Autodesk Fusion 360 part; units mm, degrees
(part 9 of 18)
  spline S49 degree 5 poles (-11.2929, 31.6454) (-11.2932, 31.6412) (-11.294, 31.6329) (-11.2951, 31.6204) (-11.2966, 31.6038) (-11.2984, 31.5831) (-11.3001, 31.5624) (-11.3019, 31.5417) (-11.3036, 31.5211) (-11.3052, 31.5006) (-11.3069, 31.48) (-11.3085, 31.4595) (-11.31, 31.4391) (-11.3116, 31.4187) (-11.3131, 31.3983) (-11.3145, 31.378) (-11.3159, 31.3577) (-11.3173, 31.3375) (-11.3187, 31.3173) (-11.32, 31.2971) (-11.3213, 31.277) (-11.3226, 31.2569) (-11.3238, 31.2369) (-11.325, 31.2169) (-11.3262, 31.1969) (-11.3273, 31.177) (-11.3284, 31.1572) (-11.3294, 31.1374) (-11.3305, 31.1176) (-11.3315, 31.0979) (-11.3324, 31.0782) (-11.3334, 31.0585) (-11.3343, 31.0389) (-11.3351, 31.0194) (-11.336, 30.9999) (-11.3368, 30.9804) (-11.3375, 30.961) (-11.3383, 30.9416) (-11.339, 30.9223) (-11.3397, 30.903) (-11.3403, 30.8838) (-11.3409, 30.8646) (-11.3415, 30.8455) (-11.342, 30.8264) (-11.3426, 30.8073) (-11.343, 30.7884) (-11.3435, 30.7694) (-11.3439, 30.7505) (-11.3443, 30.7316) (-11.3447, 30.7128) (-11.345, 30.6941) (-11.3453, 30.6754) (-11.3456, 30.6567) (-11.3458, 30.6381) (-11.3461, 30.6195) (-11.3462, 30.601) (-11.3464, 30.5826) (-11.3465, 30.5642) (-11.3466, 30.5458) (-11.3467, 30.5275) (-11.3467, 30.5092) (-11.3467, 30.491) (-11.3467, 30.4728) (-11.3466, 30.4547) (-11.3466, 30.4367) (-11.3464, 30.4187) (-11.3463, 30.4007) (-11.3461, 30.3828) (-11.3459, 30.365) (-11.3457, 30.3472) (-11.3455, 30.3294) (-11.3452, 30.3117) (-11.3449, 30.2941) (-11.3445, 30.2765) (-11.3442, 30.259) (-11.3438, 30.2415) (-11.3434, 30.2241) (-11.3429, 30.2067) (-11.3424, 30.1894) (-11.3419, 30.1722) (-11.3414, 30.155) (-11.3409, 30.1378) (-11.3403, 30.1207) (-11.3397, 30.1037) (-11.339, 30.0867) (-11.3384, 30.0698) (-11.3377, 30.053) (-11.337, 30.0362) (-11.3363, 30.0194) (-11.3355, 30.0027) (-11.3347, 29.9861) (-11.3339, 29.9695) (-11.3331, 29.953) (-11.3322, 29.9366) (-11.3313, 29.9202) (-11.3304, 29.9038) (-11.3295, 29.8876) (-11.3285, 29.8714) (-11.3275, 29.8552) (-11.3265, 29.8391) (-11.3255, 29.8231) (-11.3244, 29.8071) (-11.3234, 29.7912) (-11.3222, 29.7754) (-11.3211, 29.7596) (-11.32, 29.7439) (-11.3188, 29.7282) (-11.3176, 29.7126) (-11.3164, 29.6971) (-11.3152, 29.6817) (-11.3139, 29.6663) (-11.3126, 29.6509) (-11.3113, 29.6357) (-11.31, 29.6205) (-11.3087, 29.6053) (-11.3073, 29.5903) (-11.3059, 29.5753) (-11.3045, 29.5603) (-11.3031, 29.5454) (-11.3016, 29.5306) (-11.3002, 29.5159) (-11.2987, 29.5013) (-11.2972, 29.4867) (-11.2957, 29.4721) (-11.2941, 29.4577) (-11.2926, 29.4433) (-11.291, 29.429) (-11.2894, 29.4147) (-11.2878, 29.4006) (-11.2861, 29.3865) (-11.2845, 29.3724) (-11.2828, 29.3585) (-11.2811, 29.3446) (-11.2794, 29.3308) (-11.2777, 29.317) (-11.276, 29.3034) (-11.2742, 29.2898) (-11.2725, 29.2763) (-11.2707, 29.2628) (-11.2689, 29.2495) (-11.2671, 29.2362) (-11.2653, 29.223) (-11.2634, 29.2098) (-11.2616, 29.1968) (-11.2597, 29.1838) (-11.2578, 29.1709) (-11.2559, 29.1581) (-11.254, 29.1453) (-11.2521, 29.1327) (-11.2502, 29.1201) (-11.2482, 29.1076) (-11.2463, 29.0952) (-11.2443, 29.0829) (-11.2423, 29.0706) (-11.2403, 29.0584) (-11.2383, 29.0464) (-11.2363, 29.0344) (-11.2343, 29.0224) (-11.2323, 29.0106) (-11.2302, 28.9989) (-11.2282, 28.9872) (-11.2261, 28.9756) (-11.2241, 28.9642) (-11.222, 28.9528) (-11.2199, 28.9415) (-11.2179, 28.9302) (-11.2158, 28.9191) (-11.2137, 28.9081) (-11.2116, 28.8971) (-11.2095, 28.8863) (-11.2074, 28.8755) (-11.2053, 28.8649) (-11.2032, 28.8543) (-11.201, 28.8438) (-11.1989, 28.8335) (-11.1968, 28.8232) (-11.1947, 28.813) (-11.1926, 28.8029) (-11.1904, 28.7929) (-11.1883, 28.783) (-11.1862, 28.7733) (-11.1841, 28.7636) (-11.1819, 28.754) (-11.1798, 28.7445) (-11.1777, 28.7351) (-11.1756, 28.7259) (-11.1735, 28.7167) (-11.1714, 28.7076) (-11.1693, 28.6987) (-11.1672, 28.6898) (-11.1651, 28.6811) (-11.163, 28.6725) (-11.1609, 28.6639) (-11.1588, 28.6555) (-11.1568, 28.6473) (-11.1547, 28.6391) (-11.1527, 28.631) (-11.1507, 28.6231) (-11.1486, 28.6153) (-11.1466, 28.6075) (-11.1446, 28.6) (-11.1427, 28.5925) (-11.1407, 28.5851) (-11.1387, 28.5779) (-11.1368, 28.5708) (-11.1349, 28.5639) (-11.133, 28.557) (-11.1311, 28.5503) (-11.1293, 28.5437) (-11.1274, 28.5373) (-11.1256, 28.531) (-11.1238, 28.5248) (-11.1221, 28.5187) (-11.1203, 28.5128) (-11.1186, 28.5071) (-11.1169, 28.5014) (-11.1153, 28.496) (-11.1136, 28.4906) (-11.112, 28.4854) (-11.1105, 28.4804) (-11.1089, 28.4755) (-11.1074, 28.4708) (-11.106, 28.4662) (-11.1046, 28.4618) (-11.1032, 28.4575) (-11.1018, 28.4534) (-11.1005, 28.4495) (-11.0993, 28.4457) (-11.0981, 28.4421) (-11.0969, 28.4387) (-11.0958, 28.4354) (-11.0948, 28.4323) (-11.0937, 28.4294) (-11.0928, 28.4267) (-11.0919, 28.4242) (-11.0911, 28.4219) (-11.0903, 28.4197) (-11.0896, 28.4178) (-11.089, 28.4161) (-11.0884, 28.4145) (-11.0879, 28.4132) (-11.0876, 28.4124) (-11.0874, 28.4118) (-11.0873, 28.4115) (-11.0872, 28.4113) knots -1 -1 -1 -1 -1 -1 -0.99583333 -0.99166667 -0.9875 -0.98333333 -0.97916667 -0.975 -0.97083333 -0.96666667 -0.9625 -0.95833333 -0.95416667 -0.95 -0.94583333 -0.94166667 -0.9375 -0.93333333 -0.92916667 -0.925 -0.92083333 -0.91666667 -0.9125 -0.90833333 -0.90416667 -0.9 -0.89583333 -0.89166667 -0.8875 -0.88333333 -0.87916667 -0.875 -0.87083333 -0.86666667 -0.8625 -0.85833333 -0.85416667 -0.85 -0.84583333 -0.84166667 -0.8375 -0.83333333 -0.82916667 -0.825 -0.82083333 -0.81666667 -0.8125 -0.80833333 -0.80416667 -0.8 -0.79583333 -0.79166667 -0.7875 -0.78333333 -0.77916667 -0.775 -0.77083333 -0.76666667 -0.7625 -0.75833333 -0.75416667 -0.75 -0.74583333 -0.74166667 -0.7375 -0.73333333 -0.72916667 -0.725 -0.72083333 -0.71666667 -0.7125 -0.70833333 -0.70416667 -0.7 -0.69583333 -0.69166667 -0.6875 -0.68333333 -0.67916667 -0.675 -0.67083333 -0.66666667 -0.6625 -0.65833333 -0.65416667 -0.65 -0.64583333 -0.64166667 -0.6375 -0.63333333 -0.62916667 -0.625 -0.62083333 -0.61666667 -0.6125 -0.60833333 -0.60416667 -0.6 -0.59583333 -0.59166667 -0.5875 -0.58333333 -0.57916667 -0.575 -0.57083333 -0.56666667 -0.5625 -0.55833333 -0.55416667 -0.55 -0.54583333 -0.54166667 -0.5375 -0.53333333 -0.52916667 -0.525 -0.52083333 -0.51666667 -0.5125 -0.50833333 -0.50416667 -0.5 -0.49583333 -0.49166667 -0.4875 -0.48333333 -0.47916667 -0.475 -0.47083333 -0.46666667 -0.4625 -0.45833333 -0.45416667 -0.45 -0.44583333 -0.44166667 -0.4375 -0.43333333 -0.42916667 -0.425 -0.42083333 -0.41666667 -0.4125 -0.40833333 -0.40416667 -0.4 -0.39583333 -0.39166667 -0.3875 -0.38333333 -0.37916667 -0.375 -0.37083333 -0.36666667 -0.3625 -0.35833333 -0.35416667 -0.35 -0.34583333 -0.34166667 -0.3375 -0.33333333 -0.32916667 -0.325 -0.32083333 -0.31666667 -0.3125 -0.30833333 -0.30416667 -0.3 -0.29583333 -0.29166667 -0.2875 -0.28333333 -0.27916667 -0.275 -0.27083333 -0.26666667 -0.2625 -0.25833333 -0.25416667 -0.25 -0.24583333 -0.24166667 -0.2375 -0.23333333 -0.22916667 -0.225 -0.22083333 -0.21666667 -0.2125 -0.20833333 -0.20416667 -0.2 -0.19583333 -0.19166667 -0.1875 -0.18333333 -0.17916667 -0.175 -0.17083333 -0.16666667 -0.1625 -0.15833333 -0.15416667 -0.15 -0.14583333 -0.14166667 -0.1375 -0.13333333 -0.12916667 -0.125 -0.12083333 -0.11666667 -0.1125 -0.10833333 -0.10416667 -0.1 -0.09583333 -0.09166667 -0.0875 -0.08333333 -0.07916667 -0.075 -0.07083333 -0.06666667 -0.0625 -0.05833333 -0.05416667 -0.05 -0.04583333 -0.04166667 -0.0375 -0.03333333 -0.02916667 -0.025 -0.02083333 -0.01666667 -0.0125 -0.00833333 -0.00416667 0 0 0 0 0 0
  line L98 (-11.0872, 28.4113) -> (-11.0867, 28.41)
  line L99 (-11.0867, 28.41) -> (-10.4972, 26.8993)
  arc A50 (-10.4972, 26.8993) -> (-12.9661, 25.8001) centre (0, 0) ccw
  line L100 (-12.9661, 25.8001) -> (-13.6943, 27.2491)
  line L101 (-13.6943, 27.2491) -> (-13.6949, 27.2503)
  spline S50 degree 5 poles (-13.6949, 27.2503) (-13.695, 27.2504) (-13.6952, 27.2507) (-13.6954, 27.2513) (-13.6959, 27.2521) (-13.6965, 27.2533) (-13.6973, 27.2548) (-13.6981, 27.2564) (-13.6991, 27.2582) (-13.7002, 27.2602) (-13.7014, 27.2624) (-13.7026, 27.2647) (-13.704, 27.2673) (-13.7055, 27.2699) (-13.7071, 27.2728) (-13.7087, 27.2758) (-13.7105, 27.2789) (-13.7124, 27.2823) (-13.7144, 27.2857) (-13.7164, 27.2893) (-13.7186, 27.293) (-13.7208, 27.2969) (-13.7231, 27.3009) (-13.7256, 27.3051) (-13.7281, 27.3094) (-13.7307, 27.3138) (-13.7334, 27.3183) (-13.7362, 27.323) (-13.7391, 27.3278) (-13.742, 27.3327) (-13.7451, 27.3377) (-13.7482, 27.3428) (-13.7514, 27.3481) (-13.7547, 27.3534) (-13.7581, 27.3589) (-13.7616, 27.3645) (-13.7652, 27.3701) (-13.7688, 27.3759) (-13.7726, 27.3818) (-13.7764, 27.3878) (-13.7803, 27.3939) (-13.7843, 27.4001) (-13.7883, 27.4063) (-13.7925, 27.4127) (-13.7967, 27.4192) (-13.801, 27.4257) (-13.8054, 27.4324) (-13.8098, 27.4391) (-13.8144, 27.446) (-13.819, 27.4529) (-13.8237, 27.4599) (-13.8285, 27.4669) (-13.8334, 27.4741) (-13.8383, 27.4813) (-13.8433, 27.4887) (-13.8484, 27.4961) (-13.8536, 27.5035) (-13.8588, 27.5111) (-13.8641, 27.5187) (-13.8695, 27.5264) (-13.875, 27.5342) (-13.8806, 27.542) (-13.8862, 27.55) (-13.8919, 27.558) (-13.8977, 27.566) (-13.9035, 27.5741) (-13.9095, 27.5823) (-13.9155, 27.5906) (-13.9215, 27.5989) (-13.9277, 27.6073) (-13.9339, 27.6158) (-13.9402, 27.6243) (-13.9466, 27.6329) (-13.953, 27.6415) (-13.9595, 27.6502) (-13.9661, 27.659) (-13.9727, 27.6678) (-13.9795, 27.6767) (-13.9863, 27.6856) (-13.9931, 27.6946) (-14.0001, 27.7037) (-14.0071, 27.7128) (-14.0142, 27.7219) (-14.0213, 27.7311) (-14.0286, 27.7404) (-14.0359, 27.7497) (-14.0432, 27.7591) (-14.0507, 27.7685) (-14.0582, 27.778) (-14.0657, 27.7875) (-14.0734, 27.7971) (-14.0811, 27.8067) (-14.0889, 27.8164) (-14.0967, 27.8261) (-14.1046, 27.8358) (-14.1126, 27.8456) (-14.1207, 27.8555) (-14.1288, 27.8654) (-14.137, 27.8753) (-14.1453, 27.8853) (-14.1536, 27.8954) (-14.162, 27.9054) (-14.1704, 27.9155) (-14.179, 27.9257) (-14.1876, 27.9359) (-14.1962, 27.9461) (-14.205, 27.9564) (-14.2137, 27.9667) (-14.2226, 27.9771) (-14.2315, 27.9875) (-14.2405, 27.9979) (-14.2496, 28.0084) (-14.2587, 28.0189) (-14.2679, 28.0294) (-14.2772, 28.04) (-14.2865, 28.0506) (-14.2959, 28.0613) (-14.3053, 28.0719) (-14.3148, 28.0827) (-14.3244, 28.0934) (-14.3341, 28.1042) (-14.3438, 28.115) (-14.3536, 28.1259) (-14.3634, 28.1368) (-14.3733, 28.1477) (-14.3833, 28.1586) (-14.3933, 28.1696) (-14.4034, 28.1806) (-14.4136, 28.1916) (-14.4238, 28.2027) (-14.4341, 28.2138) (-14.4444, 28.2249) (-14.4548, 28.2361) (-14.4653, 28.2473) (-14.4758, 28.2585) (-14.4864, 28.2697) (-14.4971, 28.281) (-14.5078, 28.2923) (-14.5186, 28.3036) (-14.5295, 28.3149) (-14.5404, 28.3263) (-14.5514, 28.3377) (-14.5624, 28.3491) (-14.5735, 28.3606) (-14.5847, 28.372) (-14.5959, 28.3835) (-14.6072, 28.395) (-14.6185, 28.4066) (-14.6299, 28.4181) (-14.6414, 28.4297) (-14.6529, 28.4413) (-14.6645, 28.4529) (-14.6761, 28.4646) (-14.6878, 28.4763) (-14.6996, 28.4879) (-14.7114, 28.4997) (-14.7233, 28.5114) (-14.7353, 28.5231) (-14.7473, 28.5349) (-14.7594, 28.5467) (-14.7715, 28.5585) (-14.7837, 28.5703) (-14.7959, 28.5822) (-14.8083, 28.594) (-14.8206, 28.6059) (-14.833, 28.6178) (-14.8455, 28.6297) (-14.8581, 28.6417) (-14.8707, 28.6536) (-14.8834, 28.6656) (-14.8961, 28.6776) (-14.9089, 28.6896) (-14.9217, 28.7016) (-14.9346, 28.7136) (-14.9476, 28.7257) (-14.9606, 28.7377) (-14.9737, 28.7498) (-14.9868, 28.7619) (-15, 28.774) (-15.0132, 28.7861) (-15.0265, 28.7982) (-15.0399, 28.8104) (-15.0533, 28.8225) (-15.0668, 28.8347) (-15.0803, 28.8469) (-15.0939, 28.8591) (-15.1076, 28.8713) (-15.1213, 28.8835) (-15.1351, 28.8957) (-15.1489, 28.908) (-15.1628, 28.9202) (-15.1767, 28.9325) (-15.1907, 28.9448) (-15.2047, 28.9571) (-15.2188, 28.9693) (-15.233, 28.9816) (-15.2472, 28.994) (-15.2615, 29.0063) (-15.2758, 29.0186) (-15.2902, 29.031) (-15.3047, 29.0433) (-15.3192, 29.0557) (-15.3337, 29.068) (-15.3483, 29.0804) (-15.363, 29.0928) (-15.3777, 29.1052) (-15.3925, 29.1176) (-15.4073, 29.13) (-15.4222, 29.1424) (-15.4372, 29.1548) (-15.4522, 29.1672) (-15.4672, 29.1797) (-15.4823, 29.1921) (-15.4975, 29.2045) (-15.5127, 29.217) (-15.528, 29.2294) (-15.5433, 29.2419) (-15.5587, 29.2544) (-15.5741, 29.2668) (-15.5896, 29.2793) (-15.6052, 29.2918) (-15.6208, 29.3043) (-15.6364, 29.3168) (-15.6521, 29.3293) (-15.6679, 29.3418) (-15.6837, 29.3543) (-15.6996, 29.3668) (-15.7155, 29.3793) (-15.7315, 29.3918) (-15.7475, 29.4043) (-15.7636, 29.4168) (-15.7797, 29.4293) (-15.7959, 29.4418) (-15.8121, 29.4544) (-15.8284, 29.4669) (-15.8448, 29.4794) (-15.8612, 29.4919) (-15.8776, 29.5045) (-15.8941, 29.517) (-15.9107, 29.5295) (-15.9273, 29.5421) (-15.9406, 29.5521) (-15.9507, 29.5596) (-15.9574, 29.5646) (-15.9607, 29.5671) knots 0 0 0 0 0 0 0.00416667 0.00833333 0.0125 0.01666667 0.02083333 0.025 0.02916667 0.03333333 0.0375 0.04166667 0.04583333 0.05 0.05416667 0.05833333 0.0625 0.06666667 0.07083333 0.075 0.07916667 0.08333333 0.0875 0.09166667 0.09583333 0.1 0.10416667 0.10833333 0.1125 0.11666667 0.12083333 0.125 0.12916667 0.13333333 0.1375 0.14166667 0.14583333 0.15 0.15416667 0.15833333 0.1625 0.16666667 0.17083333 0.175 0.17916667 0.18333333 0.1875 0.19166667 0.19583333 0.2 0.20416667 0.20833333 0.2125 0.21666667 0.22083333 0.225 0.22916667 0.23333333 0.2375 0.24166667 0.24583333 0.25 0.25416667 0.25833333 0.2625 0.26666667 0.27083333 0.275 0.27916667 0.28333333 0.2875 0.29166667 0.29583333 0.3 0.30416667 0.30833333 0.3125 0.31666667 0.32083333 0.325 0.32916667 0.33333333 0.3375 0.34166667 0.34583333 0.35 0.35416667 0.35833333 0.3625 0.36666667 0.37083333 0.375 0.37916667 0.38333333 0.3875 0.39166667 0.39583333 0.4 0.40416667 0.40833333 0.4125 0.41666667 0.42083333 0.425 0.42916667 0.43333333 0.4375 0.44166667 0.44583333 0.45 0.45416667 0.45833333 0.4625 0.46666667 0.47083333 0.475 0.47916667 0.48333333 0.4875 0.49166667 0.49583333 0.5 0.50416667 0.50833333 0.5125 0.51666667 0.52083333 0.525 0.52916667 0.53333333 0.5375 0.54166667 0.54583333 0.55 0.55416667 0.55833333 0.5625 0.56666667 0.57083333 0.575 0.57916667 0.58333333 0.5875 0.59166667 0.59583333 0.6 0.60416667 0.60833333 0.6125 0.61666667 0.62083333 0.625 0.62916667 0.63333333 0.6375 0.64166667 0.64583333 0.65 0.65416667 0.65833333 0.6625 0.66666667 0.67083333 0.675 0.67916667 0.68333333 0.6875 0.69166667 0.69583333 0.7 0.70416667 0.70833333 0.7125 0.71666667 0.72083333 0.725 0.72916667 0.73333333 0.7375 0.74166667 0.74583333 0.75 0.75416667 0.75833333 0.7625 0.76666667 0.77083333 0.775 0.77916667 0.78333333 0.7875 0.79166667 0.79583333 0.8 0.80416667 0.80833333 0.8125 0.81666667 0.82083333 0.825 0.82916667 0.83333333 0.8375 0.84166667 0.84583333 0.85 0.85416667 0.85833333 0.8625 0.86666667 0.87083333 0.875 0.87916667 0.88333333 0.8875 0.89166667 0.89583333 0.9 0.90416667 0.90833333 0.9125 0.91666667 0.92083333 0.925 0.92916667 0.93333333 0.9375 0.94166667 0.94583333 0.95 0.95416667 0.95833333 0.9625 0.96666667 0.97083333 0.975 0.97916667 0.98333333 0.9875 0.99166667 0.99583333 1 1 1 1 1 1
  arc A51 (-15.9607, 29.5671) -> (-17.6255, 28.606) centre (0, 0) ccw
  spline S51 degree 5 poles (-17.6255, 28.606) (-17.625, 28.6018) (-17.624, 28.5935) (-17.6225, 28.5811) (-17.6205, 28.5645) (-17.618, 28.5438) (-17.6154, 28.5232) (-17.6128, 28.5027) (-17.6102, 28.4822) (-17.6075, 28.4617) (-17.6049, 28.4413) (-17.6022, 28.4209) (-17.5994, 28.4006) (-17.5967, 28.3803) (-17.5939, 28.3601) (-17.5911, 28.3399) (-17.5883, 28.3197) (-17.5854, 28.2996) (-17.5826, 28.2796) (-17.5797, 28.2596) (-17.5768, 28.2397) (-17.5738, 28.2198) (-17.5709, 28.1999) (-17.5679, 28.1801) (-17.5649, 28.1604) (-17.5618, 28.1407) (-17.5588, 28.121) (-17.5557, 28.1014) (-17.5526, 28.0819) (-17.5494, 28.0624) (-17.5463, 28.0429) (-17.5431, 28.0235) (-17.5399, 28.0041) (-17.5367, 27.9848) (-17.5335, 27.9656) (-17.5302, 27.9464) (-17.5269, 27.9272) (-17.5236, 27.9081) (-17.5203, 27.8891) (-17.517, 27.8701) (-17.5136, 27.8511) (-17.5102, 27.8322) (-17.5068, 27.8134) (-17.5034, 27.7946) (-17.4999, 27.7759) (-17.4964, 27.7572) (-17.4929, 27.7386) (-17.4894, 27.72) (-17.4859, 27.7015) (-17.4823, 27.683) (-17.4788, 27.6646) (-17.4752, 27.6462) (-17.4716, 27.6279) (-17.4679, 27.6097) (-17.4643, 27.5915) (-17.4606, 27.5733) (-17.4569, 27.5552) (-17.4532, 27.5372) (-17.4495, 27.5192) (-17.4457, 27.5013) (-17.442, 27.4834) (-17.4382, 27.4656) (-17.4344, 27.4478) (-17.4306, 27.4301) (-17.4267, 27.4125) (-17.4229, 27.3949) (-17.419, 27.3774) (-17.4151, 27.3599) (-17.4112, 27.3425) (-17.4073, 27.3251) (-17.4034, 27.3078) (-17.3994, 27.2906) (-17.3955, 27.2734) (-17.3915, 27.2562) (-17.3875, 27.2392) (-17.3835, 27.2222) (-17.3794, 27.2052) (-17.3754, 27.1883) (-17.3713, 27.1715) (-17.3672, 27.1547) (-17.3632, 27.138) (-17.359, 27.1213) (-17.3549, 27.1048) (-17.3508, 27.0882) (-17.3466, 27.0717) (-17.3425, 27.0553) (-17.3383, 27.039) (-17.3341, 27.0227) (-17.3299, 27.0065) (-17.3257, 26.9903) (-17.3215, 26.9742) (-17.3172, 26.9582) (-17.313, 26.9422) (-17.3087, 26.9263) (-17.3044, 26.9104) (-17.3002, 26.8947) (-17.2959, 26.8789) (-17.2916, 26.8633) (-17.2872, 26.8477) (-17.2829, 26.8322) (-17.2786, 26.8167) (-17.2742, 26.8013) (-17.2699, 26.786) (-17.2655, 26.7707) (-17.2611, 26.7555) (-17.2567, 26.7404) (-17.2523, 26.7253) (-17.2479, 26.7103) (-17.2435, 26.6954) (-17.2391, 26.6805) (-17.2346, 26.6657) (-17.2302, 26.651) (-17.2258, 26.6363) (-17.2213, 26.6217) (-17.2168, 26.6072) (-17.2124, 26.5927) (-17.2079, 26.5783) (-17.2034, 26.564) (-17.1989, 26.5498) (-17.1944, 26.5356) (-17.1899, 26.5215) (-17.1854, 26.5074) (-17.1809, 26.4935) (-17.1764, 26.4796) (-17.1719, 26.4658) (-17.1674, 26.452) (-17.1629, 26.4384) (-17.1584, 26.4247) (-17.1538, 26.4112) (-17.1493, 26.3978) (-17.1448, 26.3844) (-17.1402, 26.3711) (-17.1357, 26.3578) (-17.1312, 26.3447) (-17.1266, 26.3316) (-17.1221, 26.3186) (-17.1175, 26.3057) (-17.113, 26.2928) (-17.1085, 26.2801) (-17.1039, 26.2674) (-17.0994, 26.2547) (-17.0949, 26.2422) (-17.0903, 26.2297) (-17.0858, 26.2173) (-17.0813, 26.205) (-17.0768, 26.1928) (-17.0723, 26.1807) (-17.0677, 26.1686) (-17.0632, 26.1566) (-17.0587, 26.1447) (-17.0542, 26.1329) (-17.0497, 26.1212) (-17.0452, 26.1095) (-17.0408, 26.0979) (-17.0363, 26.0864) (-17.0318, 26.075) (-17.0274, 26.0637) (-17.0229, 26.0525) (-17.0185, 26.0413) (-17.014, 26.0303) (-17.0096, 26.0193) (-17.0052, 26.0084) (-17.0008, 25.9976) (-16.9964, 25.9869) (-16.992, 25.9763) (-16.9877, 25.9657) (-16.9833, 25.9553) (-16.979, 25.9449) (-16.9746, 25.9347) (-16.9703, 25.9245) (-16.966, 25.9144) (-16.9618, 25.9044) (-16.9575, 25.8945) (-16.9532, 25.8847) (-16.949, 25.875) (-16.9448, 25.8654) (-16.9406, 25.8559) (-16.9364, 25.8464) (-16.9323, 25.8371) (-16.9281, 25.8279) (-16.924, 25.8188) (-16.9199, 25.8097) (-16.9159, 25.8008) (-16.9118, 25.792) (-16.9078, 25.7832) (-16.9038, 25.7746) (-16.8998, 25.7661) (-16.8959, 25.7576) (-16.892, 25.7493) (-16.8881, 25.7411) (-16.8842, 25.733) (-16.8804, 25.725) (-16.8766, 25.7171) (-16.8728, 25.7093) (-16.8691, 25.7016) (-16.8654, 25.6941) (-16.8617, 25.6866) (-16.8581, 25.6792) (-16.8545, 25.672) (-16.8509, 25.6649) (-16.8474, 25.6579) (-16.8439, 25.651) (-16.8404, 25.6442) (-16.837, 25.6376) (-16.8337, 25.631) (-16.8303, 25.6246) (-16.8271, 25.6183) (-16.8238, 25.6121) (-16.8206, 25.6061) (-16.8175, 25.6001) (-16.8144, 25.5943) (-16.8114, 25.5887) (-16.8084, 25.5831) (-16.8055, 25.5777) (-16.8026, 25.5724) (-16.7998, 25.5673) (-16.797, 25.5623) (-16.7943, 25.5574) (-16.7917, 25.5526) (-16.7891, 25.548) (-16.7866, 25.5436) (-16.7841, 25.5392) (-16.7817, 25.5351) (-16.7794, 25.531) (-16.7772, 25.5271) (-16.775, 25.5234) (-16.7729, 25.5198) (-16.7709, 25.5164) (-16.769, 25.5131) (-16.7672, 25.51) (-16.7654, 25.5071) (-16.7637, 25.5043) (-16.7621, 25.5017) (-16.7606, 25.4992) (-16.7593, 25.4969) (-16.758, 25.4948) (-16.7568, 25.4929) (-16.7557, 25.4911) (-16.7547, 25.4896) (-16.7538, 25.4882) (-16.7531, 25.487) (-16.7526, 25.4862) (-16.7523, 25.4857) (-16.7521, 25.4854) (-16.752, 25.4853) knots -1 -1 -1 -1 -1 -1 -0.99583333 -0.99166667 -0.9875 -0.98333333 -0.97916667 -0.975 -0.97083333 -0.96666667 -0.9625 -0.95833333 -0.95416667 -0.95 -0.94583333 -0.94166667 -0.9375 -0.93333333 -0.92916667 -0.925 -0.92083333 -0.91666667 -0.9125 -0.90833333 -0.90416667 -0.9 -0.89583333 -0.89166667 -0.8875 -0.88333333 -0.87916667 -0.875 -0.87083333 -0.86666667 -0.8625 -0.85833333 -0.85416667 -0.85 -0.84583333 -0.84166667 -0.8375 -0.83333333 -0.82916667 -0.825 -0.82083333 -0.81666667 -0.8125 -0.80833333 -0.80416667 -0.8 -0.79583333 -0.79166667 -0.7875 -0.78333333 -0.77916667 -0.775 -0.77083333 -0.76666667 -0.7625 -0.75833333 -0.75416667 -0.75 -0.74583333 -0.74166667 -0.7375 -0.73333333 -0.72916667 -0.725 -0.72083333 -0.71666667 -0.7125 -0.70833333 -0.70416667 -0.7 -0.69583333 -0.69166667 -0.6875 -0.68333333 -0.67916667 -0.675 -0.67083333 -0.66666667 -0.6625 -0.65833333 -0.65416667 -0.65 -0.64583333 -0.64166667 -0.6375 -0.63333333 -0.62916667 -0.625 -0.62083333 -0.61666667 -0.6125 -0.60833333 -0.60416667 -0.6 -0.59583333 -0.59166667 -0.5875 -0.58333333 -0.57916667 -0.575 -0.57083333 -0.56666667 -0.5625 -0.55833333 -0.55416667 -0.55 -0.54583333 -0.54166667 -0.5375 -0.53333333 -0.52916667 -0.525 -0.52083333 -0.51666667 -0.5125 -0.50833333 -0.50416667 -0.5 -0.49583333 -0.49166667 -0.4875 -0.48333333 -0.47916667 -0.475 -0.47083333 -0.46666667 -0.4625 -0.45833333 -0.45416667 -0.45 -0.44583333 -0.44166667 -0.4375 -0.43333333 -0.42916667 -0.425 -0.42083333 -0.41666667 -0.4125 -0.40833333 -0.40416667 -0.4 -0.39583333 -0.39166667 -0.3875 -0.38333333 -0.37916667 -0.375 -0.37083333 -0.36666667 -0.3625 -0.35833333 -0.35416667 -0.35 -0.34583333 -0.34166667 -0.3375 -0.33333333 -0.32916667 -0.325 -0.32083333 -0.31666667 -0.3125 -0.30833333 -0.30416667 -0.3 -0.29583333 -0.29166667 -0.2875 -0.28333333 -0.27916667 -0.275 -0.27083333 -0.26666667 -0.2625 -0.25833333 -0.25416667 -0.25 -0.24583333 -0.24166667 -0.2375 -0.23333333 -0.22916667 -0.225 -0.22083333 -0.21666667 -0.2125 -0.20833333 -0.20416667 -0.2 -0.19583333 -0.19166667 -0.1875 -0.18333333 -0.17916667 -0.175 -0.17083333 -0.16666667 -0.1625 -0.15833333 -0.15416667 -0.15 -0.14583333 -0.14166667 -0.1375 -0.13333333 -0.12916667 -0.125 -0.12083333 -0.11666667 -0.1125 -0.10833333 -0.10416667 -0.1 -0.09583333 -0.09166667 -0.0875 -0.08333333 -0.07916667 -0.075 -0.07083333 -0.06666667 -0.0625 -0.05833333 -0.05416667 -0.05 -0.04583333 -0.04166667 -0.0375 -0.03333333 -0.02916667 -0.025 -0.02083333 -0.01666667 -0.0125 -0.00833333 -0.00416667 0 0 0 0 0 0
  line L102 (-16.752, 25.4853) -> (-16.7512, 25.4842)
  line L103 (-16.7512, 25.4842) -> (-15.8605, 24.129)
  arc A52 (-15.8605, 24.129) -> (-18.0469, 22.5405) centre (0, 0) ccw
  line L104 (-18.0469, 22.5405) -> (-19.0605, 23.8064)
  line L105 (-19.0605, 23.8064) -> (-19.0613, 23.8075)
  spline S52 degree 5 poles (-19.0613, 23.8075) (-19.0614, 23.8076) (-19.0616, 23.8079) (-19.062, 23.8083) (-19.0626, 23.809) (-19.0635, 23.8101) (-19.0645, 23.8114) (-19.0657, 23.8128) (-19.0671, 23.8144) (-19.0685, 23.8161) (-19.0701, 23.818) (-19.0719, 23.82) (-19.0737, 23.8222) (-19.0757, 23.8245) (-19.0779, 23.827) (-19.0801, 23.8295) (-19.0825, 23.8323) (-19.085, 23.8351) (-19.0877, 23.8381) (-19.0904, 23.8412) (-19.0933, 23.8444) (-19.0963, 23.8477) (-19.0994, 23.8512) (-19.1027, 23.8547) (-19.106, 23.8584) (-19.1095, 23.8621) (-19.1131, 23.866) (-19.1168, 23.87) (-19.1206, 23.8741) (-19.1245, 23.8783) (-19.1285, 23.8825) (-19.1327, 23.8869) (-19.1369, 23.8914) (-19.1413, 23.8959) (-19.1457, 23.9005) (-19.1503, 23.9053) (-19.155, 23.9101) (-19.1597, 23.915) (-19.1646, 23.92) (-19.1696, 23.925) (-19.1747, 23.9302) (-19.1798, 23.9354) (-19.1851, 23.9407) (-19.1905, 23.9461) (-19.196, 23.9515) (-19.2015, 23.957) (-19.2072, 23.9626) (-19.213, 23.9683) (-19.2188, 23.974) (-19.2248, 23.9798) (-19.2309, 23.9857) (-19.237, 23.9916) (-19.2433, 23.9976) (-19.2496, 24.0037) (-19.256, 24.0098) (-19.2625, 24.016) (-19.2692, 24.0222) (-19.2759, 24.0285) (-19.2826, 24.0348) (-19.2895, 24.0413) (-19.2965, 24.0477) (-19.3036, 24.0542) (-19.3107, 24.0608) (-19.318, 24.0675) (-19.3253, 24.0741) (-19.3327, 24.0809) (-19.3402, 24.0877) (-19.3478, 24.0945) (-19.3554, 24.1014) (-19.3632, 24.1083) (-19.371, 24.1153) (-19.379, 24.1223) (-19.387, 24.1294) (-19.3951, 24.1365) (-19.4033, 24.1436) (-19.4115, 24.1509) (-19.4199, 24.1581) (-19.4283, 24.1654) (-19.4368, 24.1727) (-19.4454, 24.1801) (-19.4541, 24.1875) (-19.4628, 24.1949) (-19.4717, 24.2024) (-19.4806, 24.2099) (-19.4896, 24.2175) (-19.4986, 24.2251) (-19.5078, 24.2327) (-19.517, 24.2404) (-19.5263, 24.2481) (-19.5357, 24.2559) (-19.5452, 24.2636) (-19.5547, 24.2714) (-19.5643, 24.2793) (-19.574, 24.2871) (-19.5838, 24.295) (-19.5937, 24.303) (-19.6036, 24.3109) (-19.6136, 24.3189) (-19.6237, 24.3269) (-19.6338, 24.335) (-19.6441, 24.3431) (-19.6544, 24.3512) (-19.6647, 24.3593) (-19.6752, 24.3675) (-19.6857, 24.3757) (-19.6963, 24.3839) (-19.707, 24.3921) (-19.7178, 24.4004) (-19.7286, 24.4087) (-19.7395, 24.417) (-19.7504, 24.4253) (-19.7615, 24.4337) (-19.7726, 24.442) (-19.7838, 24.4504) (-19.795, 24.4589) (-19.8063, 24.4673) (-19.8177, 24.4758) (-19.8292, 24.4843) (-19.8407, 24.4928) (-19.8524, 24.5013) (-19.864, 24.5098) (-19.8758, 24.5184) (-19.8876, 24.527) (-19.8995, 24.5356) (-19.9114, 24.5442) (-19.9235, 24.5528) (-19.9356, 24.5615) (-19.9477, 24.5702) (-19.96, 24.5788) (-19.9723, 24.5875) (-19.9846, 24.5963) (-19.9971, 24.605) (-20.0096, 24.6137) (-20.0221, 24.6225) (-20.0348, 24.6313) (-20.0475, 24.6401) (-20.0603, 24.6489) (-20.0731, 24.6577) (-20.086, 24.6665) (-20.099, 24.6753) (-20.112, 24.6842) (-20.1251, 24.693) (-20.1383, 24.7019) (-20.1515, 24.7108) (-20.1648, 24.7197) (-20.1782, 24.7286) (-20.1916, 24.7375) (-20.2051, 24.7465) (-20.2187, 24.7554) (-20.2323, 24.7643) (-20.246, 24.7733) (-20.2597, 24.7823) (-20.2735, 24.7912) (-20.2874, 24.8002) (-20.3014, 24.8092) (-20.3154, 24.8182) (-20.3294, 24.8272) (-20.3436, 24.8362) (-20.3578, 24.8452) (-20.372, 24.8542) (-20.3864, 24.8633) (-20.4007, 24.8723) (-20.4152, 24.8813) (-20.4297, 24.8904) (-20.4443, 24.8994) (-20.4589, 24.9085) (-20.4736, 24.9176) (-20.4883, 24.9266) (-20.5032, 24.9357) (-20.518, 24.9448) (-20.533, 24.9538) (-20.548, 24.9629) (-20.563, 24.972) (-20.5781, 24.9811) (-20.5933, 24.9902) (-20.6086, 24.9993) (-20.6239, 25.0084) (-20.6392, 25.0174) (-20.6546, 25.0265) (-20.6701, 25.0356) (-20.6857, 25.0447) (-20.7013, 25.0538) (-20.7169, 25.0629) (-20.7326, 25.072) (-20.7484, 25.0811) (-20.7642, 25.0902) (-20.7801, 25.0993) (-20.7961, 25.1084) (-20.8121, 25.1175) (-20.8281, 25.1266) (-20.8443, 25.1357) (-20.8605, 25.1448) (-20.8767, 25.1539) (-20.893, 25.163) (-20.9093, 25.1721) (-20.9258, 25.1812) (-20.9422, 25.1903) (-20.9588, 25.1994) (-20.9753, 25.2085) (-20.992, 25.2175) (-21.0087, 25.2266) (-21.0254, 25.2357) (-21.0422, 25.2448) (-21.0591, 25.2538) (-21.076, 25.2629) (-21.093, 25.2719) (-21.11, 25.281) (-21.1271, 25.29) (-21.1443, 25.2991) (-21.1615, 25.3081) (-21.1787, 25.3172) (-21.196, 25.3262) (-21.2134, 25.3352) (-21.2308, 25.3442) (-21.2483, 25.3533) (-21.2658, 25.3623) (-21.2834, 25.3713) (-21.301, 25.3803) (-21.3187, 25.3892) (-21.3365, 25.3982) (-21.3543, 25.4072) (-21.3721, 25.4162) (-21.39, 25.4251) (-21.408, 25.4341) (-21.426, 25.443) (-21.4441, 25.452) (-21.4622, 25.4609) (-21.4804, 25.4698) (-21.4986, 25.4787) (-21.5169, 25.4876) (-21.5352, 25.4965) (-21.5536, 25.5054) (-21.572, 25.5143) (-21.5905, 25.5232) (-21.6091, 25.5321) (-21.6277, 25.5409) (-21.6463, 25.5498) (-21.665, 25.5586) (-21.6838, 25.5674) (-21.7026, 25.5762) (-21.7214, 25.585) (-21.7365, 25.5921) (-21.7479, 25.5973) (-21.7555, 25.6009) (-21.7593, 25.6026) knots 0 0 0 0 0 0 0.00416667 0.00833333 0.0125 0.01666667 0.02083333 0.025 0.02916667 0.03333333 0.0375 0.04166667 0.04583333 0.05 0.05416667 0.05833333 0.0625 0.06666667 0.07083333 0.075 0.07916667 0.08333333 0.0875 0.09166667 0.09583333 0.1 0.10416667 0.10833333 0.1125 0.11666667 0.12083333 0.125 0.12916667 0.13333333 0.1375 0.14166667 0.14583333 0.15 0.15416667 0.15833333 0.1625 0.16666667 0.17083333 0.175 0.17916667 0.18333333 0.1875 0.19166667 0.19583333 0.2 0.20416667 0.20833333 0.2125 0.21666667 0.22083333 0.225 0.22916667 0.23333333 0.2375 0.24166667 0.24583333 0.25 0.25416667 0.25833333 0.2625 0.26666667 0.27083333 0.275 0.27916667 0.28333333 0.2875 0.29166667 0.29583333 0.3 0.30416667 0.30833333 0.3125 0.31666667 0.32083333 0.325 0.32916667 0.33333333 0.3375 0.34166667 0.34583333 0.35 0.35416667 0.35833333 0.3625 0.36666667 0.37083333 0.375 0.37916667 0.38333333 0.3875 0.39166667 0.39583333 0.4 0.40416667 0.40833333 0.4125 0.41666667 0.42083333 0.425 0.42916667 0.43333333 0.4375 0.44166667 0.44583333 0.45 0.45416667 0.45833333 0.4625 0.46666667 0.47083333 0.475 0.47916667 0.48333333 0.4875 0.49166667 0.49583333 0.5 0.50416667 0.50833333 0.5125 0.51666667 0.52083333 0.525 0.52916667 0.53333333 0.5375 0.54166667 0.54583333 0.55 0.55416667 0.55833333 0.5625 0.56666667 0.57083333 0.575 0.57916667 0.58333333 0.5875 0.59166667 0.59583333 0.6 0.60416667 0.60833333 0.6125 0.61666667 0.62083333 0.625 0.62916667 0.63333333 0.6375 0.64166667 0.64583333 0.65 0.65416667 0.65833333 0.6625 0.66666667 0.67083333 0.675 0.67916667 0.68333333 0.6875 0.69166667 0.69583333 0.7 0.70416667 0.70833333 0.7125 0.71666667 0.72083333 0.725 0.72916667 0.73333333 0.7375 0.74166667 0.74583333 0.75 0.75416667 0.75833333 0.7625 0.76666667 0.77083333 0.775 0.77916667 0.78333333 0.7875 0.79166667 0.79583333 0.8 0.80416667 0.80833333 0.8125 0.81666667 0.82083333 0.825 0.82916667 0.83333333 0.8375 0.84166667 0.84583333 0.85 0.85416667 0.85833333 0.8625 0.86666667 0.87083333 0.875 0.87916667 0.88333333 0.8875 0.89166667 0.89583333 0.9 0.90416667 0.90833333 0.9125 0.91666667 0.92083333 0.925 0.92916667 0.93333333 0.9375 0.94166667 0.94583333 0.95 0.95416667 0.95833333 0.9625 0.96666667 0.97083333 0.975 0.97916667 0.98333333 0.9875 0.99166667 0.99583333 1 1 1 1 1 1
  arc A53 (-21.7593, 25.6026) -> (-23.1879, 24.3163) centre (0, 0) ccw
  spline S53 degree 5 poles (-23.1879, 24.3163) (-23.1865, 24.3123) (-23.1838, 24.3044) (-23.1798, 24.2926) (-23.1744, 24.2768) (-23.1676, 24.2571) (-23.1608, 24.2375) (-23.154, 24.2179) (-23.1471, 24.1984) (-23.1403, 24.1789) (-23.1334, 24.1595) (-23.1265, 24.1401) (-23.1197, 24.1208) (-23.1128, 24.1016) (-23.1058, 24.0823) (-23.0989, 24.0632) (-23.092, 24.0441) (-23.085, 24.025) (-23.078, 24.006) (-23.071, 23.9871) (-23.064, 23.9681) (-23.057, 23.9493) (-23.05, 23.9305) (-23.0429, 23.9118) (-23.0359, 23.8931) (-23.0288, 23.8744) (-23.0217, 23.8558) (-23.0147, 23.8373) (-23.0076, 23.8188) (-23.0004, 23.8004) (-22.9933, 23.782) (-22.9862, 23.7637) (-22.979, 23.7454) (-22.9719, 23.7272) (-22.9647, 23.7091) (-22.9575, 23.691) (-22.9503, 23.6729) (-22.9431, 23.6549) (-22.9359, 23.637) (-22.9287, 23.6191) (-22.9215, 23.6012) (-22.9142, 23.5835) (-22.907, 23.5658) (-22.8997, 23.5481) (-22.8924, 23.5305) (-22.8851, 23.5129) (-22.8778, 23.4954) (-22.8705, 23.478) (-22.8632, 23.4606) (-22.8559, 23.4433) (-22.8486, 23.426) (-22.8413, 23.4088) (-22.8339, 23.3916) (-22.8266, 23.3745) (-22.8192, 23.3575) (-22.8119, 23.3405) (-22.8045, 23.3236) (-22.7971, 23.3067) (-22.7897, 23.2899) (-22.7823, 23.2731) (-22.7749, 23.2564) (-22.7675, 23.2398) (-22.7601, 23.2232) (-22.7527, 23.2067) (-22.7453, 23.1902) (-22.7379, 23.1738) (-22.7304, 23.1575) (-22.723, 23.1412) (-22.7156, 23.125) (-22.7081, 23.1088) (-22.7007, 23.0927) (-22.6932, 23.0766) (-22.6858, 23.0607) (-22.6783, 23.0447) (-22.6709, 23.0289) (-22.6634, 23.0131) (-22.6559, 22.9973) (-22.6485, 22.9816) (-22.641, 22.966) (-22.6335, 22.9505) (-22.626, 22.935) (-22.6186, 22.9195) (-22.6111, 22.9042) (-22.6036, 22.8888) (-22.5961, 22.8736) (-22.5886, 22.8584) (-22.5811, 22.8433) (-22.5737, 22.8282) (-22.5662, 22.8132) (-22.5587, 22.7983) (-22.5512, 22.7834) (-22.5437, 22.7686) (-22.5363, 22.7539) (-22.5288, 22.7392) (-22.5213, 22.7246) (-22.5138, 22.71) (-22.5064, 22.6955) (-22.4989, 22.6811) (-22.4914, 22.6668) (-22.484, 22.6525) (-22.4765, 22.6383) (-22.469, 22.6241) (-22.4616, 22.61) (-22.4541, 22.596) (-22.4467, 22.582) (-22.4392, 22.5681) (-22.4318, 22.5543) (-22.4244, 22.5406) (-22.417, 22.5269) (-22.4095, 22.5132) (-22.4021, 22.4997) (-22.3947, 22.4862) (-22.3873, 22.4728) (-22.3799, 22.4594) (-22.3725, 22.4462) (-22.3652, 22.4329) (-22.3578, 22.4198) (-22.3504, 22.4067) (-22.3431, 22.3937) (-22.3358, 22.3808) (-22.3284, 22.3679) (-22.3211, 22.3551) (-22.3138, 22.3424) (-22.3065, 22.3298) (-22.2992, 22.3172) (-22.2919, 22.3047) (-22.2847, 22.2922) (-22.2774, 22.2799) (-22.2702, 22.2676) (-22.2629, 22.2554) (-22.2557, 22.2432) (-22.2485, 22.2312) (-22.2413, 22.2192) (-22.2342, 22.2072) (-22.227, 22.1954) (-22.2199, 22.1836) (-22.2127, 22.1719) (-22.2056, 22.1603) (-22.1985, 22.1487) (-22.1915, 22.1372) (-22.1844, 22.1258) (-22.1774, 22.1145) (-22.1703, 22.1033) (-22.1633, 22.0921) (-22.1564, 22.081) (-22.1494, 22.07) (-22.1424, 22.059) (-22.1355, 22.0482) (-22.1286, 22.0374) (-22.1217, 22.0267) (-22.1149, 22.0161) (-22.108, 22.0055) (-22.1012, 21.995) (-22.0944, 21.9847) (-22.0877, 21.9743) (-22.0809, 21.9641) (-22.0742, 21.954) (-22.0675, 21.9439) (-22.0609, 21.9339) (-22.0542, 21.924) (-22.0476, 21.9142) (-22.041, 21.9045) (-22.0345, 21.8948) (-22.028, 21.8853) (-22.0215, 21.8758) (-22.015, 21.8664) (-22.0086, 21.8571) (-22.0022, 21.8478) (-21.9958, 21.8387) (-21.9895, 21.8296) (-21.9832, 21.8207) (-21.9769, 21.8118) (-21.9707, 21.803) (-21.9645, 21.7943) (-21.9583, 21.7857) (-21.9522, 21.7771) (-21.9461, 21.7687) (-21.9401, 21.7603) (-21.9341, 21.7521) (-21.9281, 21.7439) (-21.9222, 21.7358) (-21.9163, 21.7279) (-21.9105, 21.72) (-21.9047, 21.7122) (-21.899, 21.7045) (-21.8933, 21.6969) (-21.8876, 21.6893) (-21.882, 21.6819) (-21.8764, 21.6746) (-21.8709, 21.6674) (-21.8654, 21.6602) (-21.86, 21.6532) (-21.8547, 21.6463) (-21.8494, 21.6394) (-21.8441, 21.6327) (-21.8389, 21.6261) (-21.8338, 21.6195) (-21.8287, 21.6131) (-21.8237, 21.6068) (-21.8187, 21.6005) (-21.8138, 21.5944) (-21.8089, 21.5884) (-21.8042, 21.5825) (-21.7994, 21.5767) (-21.7948, 21.571) (-21.7902, 21.5654) (-21.7857, 21.5599) (-21.7812, 21.5546) (-21.7769, 21.5493) (-21.7726, 21.5442) (-21.7683, 21.5391) (-21.7642, 21.5342) (-21.7601, 21.5294) (-21.7561, 21.5247) (-21.7522, 21.5201) (-21.7484, 21.5157) (-21.7446, 21.5114) (-21.741, 21.5071) (-21.7374, 21.5031) (-21.7339, 21.4991) (-21.7305, 21.4952) (-21.7273, 21.4915) (-21.7241, 21.4879) (-21.721, 21.4845) (-21.718, 21.4811) (-21.7151, 21.4779) (-21.7123, 21.4749) (-21.7096, 21.4719) (-21.707, 21.4691) (-21.7046, 21.4665) (-21.7022, 21.464) (-21.7, 21.4616) (-21.6979, 21.4593) (-21.696, 21.4573) (-21.6941, 21.4553) (-21.6924, 21.4535) (-21.6909, 21.4519) (-21.6894, 21.4504) (-21.6881, 21.4491) (-21.687, 21.4479) (-21.686, 21.4469) (-21.6854, 21.4462) (-21.685, 21.4458) (-21.6847, 21.4456) (-21.6846, 21.4454) knots -1 -1 -1 -1 -1 -1 -0.99583333 -0.99166667 -0.9875 -0.98333333 -0.97916667 -0.975 -0.97083333 -0.96666667 -0.9625 -0.95833333 -0.95416667 -0.95 -0.94583333 -0.94166667 -0.9375 -0.93333333 -0.92916667 -0.925 -0.92083333 -0.91666667 -0.9125 -0.90833333 -0.90416667 -0.9 -0.89583333 -0.89166667 -0.8875 -0.88333333 -0.87916667 -0.875 -0.87083333 -0.86666667 -0.8625 -0.85833333 -0.85416667 -0.85 -0.84583333 -0.84166667 -0.8375 -0.83333333 -0.82916667 -0.825 -0.82083333 -0.81666667 -0.8125 -0.80833333 -0.80416667 -0.8 -0.79583333 -0.79166667 -0.7875 -0.78333333 -0.77916667 -0.775 -0.77083333 -0.76666667 -0.7625 -0.75833333 -0.75416667 -0.75 -0.74583333 -0.74166667 -0.7375 -0.73333333 -0.72916667 -0.725 -0.72083333 -0.71666667 -0.7125 -0.70833333 -0.70416667 -0.7 -0.69583333 -0.69166667 -0.6875 -0.68333333 -0.67916667 -0.675 -0.67083333 -0.66666667 -0.6625 -0.65833333 -0.65416667 -0.65 -0.64583333 -0.64166667 -0.6375 -0.63333333 -0.62916667 -0.625 -0.62083333 -0.61666667 -0.6125 -0.60833333 -0.60416667 -0.6 -0.59583333 -0.59166667 -0.5875 -0.58333333 -0.57916667 -0.575 -0.57083333 -0.56666667 -0.5625 -0.55833333 -0.55416667 -0.55 -0.54583333 -0.54166667 -0.5375 -0.53333333 -0.52916667 -0.525 -0.52083333 -0.51666667 -0.5125 -0.50833333 -0.50416667 -0.5 -0.49583333 -0.49166667 -0.4875 -0.48333333 -0.47916667 -0.475 -0.47083333 -0.46666667 -0.4625 -0.45833333 -0.45416667 -0.45 -0.44583333 -0.44166667 -0.4375 -0.43333333 -0.42916667 -0.425 -0.42083333 -0.41666667 -0.4125 -0.40833333 -0.40416667 -0.4 -0.39583333 -0.39166667 -0.3875 -0.38333333 -0.37916667 -0.375 -0.37083333 -0.36666667 -0.3625 -0.35833333 -0.35416667 -0.35 -0.34583333 -0.34166667 -0.3375 -0.33333333 -0.32916667 -0.325 -0.32083333 -0.31666667 -0.3125 -0.30833333 -0.30416667 -0.3 -0.29583333 -0.29166667 -0.2875 -0.28333333 -0.27916667 -0.275 -0.27083333 -0.26666667 -0.2625 -0.25833333 -0.25416667 -0.25 -0.24583333 -0.24166667 -0.2375 -0.23333333 -0.22916667 -0.225 -0.22083333 -0.21666667 -0.2125 -0.20833333 -0.20416667 -0.2 -0.19583333 -0.19166667 -0.1875 -0.18333333 -0.17916667 -0.175 -0.17083333 -0.16666667 -0.1625 -0.15833333 -0.15416667 -0.15 -0.14583333 -0.14166667 -0.1375 -0.13333333 -0.12916667 -0.125 -0.12083333 -0.11666667 -0.1125 -0.10833333 -0.10416667 -0.1 -0.09583333 -0.09166667 -0.0875 -0.08333333 -0.07916667 -0.075 -0.07083333 -0.06666667 -0.0625 -0.05833333 -0.05416667 -0.05 -0.04583333 -0.04166667 -0.0375 -0.03333333 -0.02916667 -0.025 -0.02083333 -0.01666667 -0.0125 -0.00833333 -0.00416667 0 0 0 0 0 0
  line L106 (-21.6846, 21.4454) -> (-21.6836, 21.4445)
  line L107 (-21.6836, 21.4445) -> (-20.5306, 20.3042)
  arc A54 (-20.5306, 20.3042) -> (-22.339, 18.2958) centre (0, 0) ccw
  line L108 (-22.339, 18.2958) -> (-23.5936, 19.3233)
  line L109 (-23.5936, 19.3233) -> (-23.5946, 19.3241)
  spline S54 degree 5 poles (-23.5946, 19.3241) (-23.5948, 19.3242) (-23.595, 19.3245) (-23.5955, 19.3248) (-23.5962, 19.3254) (-23.5973, 19.3263) (-23.5986, 19.3273) (-23.6001, 19.3284) (-23.6017, 19.3297) (-23.6035, 19.3311) (-23.6054, 19.3326) (-23.6076, 19.3342) (-23.6098, 19.336) (-23.6123, 19.3378) (-23.6149, 19.3398) (-23.6176, 19.3418) (-23.6205, 19.344) (-23.6236, 19.3462) (-23.6268, 19.3486) (-23.6301, 19.3511) (-23.6336, 19.3536) (-23.6372, 19.3562) (-23.641, 19.3589) (-23.6449, 19.3618) (-23.649, 19.3646) (-23.6531, 19.3676) (-23.6574, 19.3707) (-23.6619, 19.3738) (-23.6665, 19.377) (-23.6712, 19.3802) (-23.676, 19.3836) (-23.6809, 19.387) (-23.686, 19.3905) (-23.6912, 19.394) (-23.6965, 19.3976) (-23.702, 19.4013) (-23.7076, 19.4051) (-23.7132, 19.4089) (-23.7191, 19.4127) (-23.725, 19.4166) (-23.731, 19.4206) (-23.7372, 19.4246) (-23.7434, 19.4287) (-23.7498, 19.4329) (-23.7563, 19.4371) (-23.7629, 19.4413) (-23.7696, 19.4456) (-23.7764, 19.4499) (-23.7834, 19.4543) (-23.7904, 19.4587) (-23.7975, 19.4632) (-23.8048, 19.4677) (-23.8121, 19.4723) (-23.8196, 19.4769) (-23.8271, 19.4816) (-23.8348, 19.4862) (-23.8426, 19.491) (-23.8504, 19.4957) (-23.8584, 19.5005) (-23.8665, 19.5054) (-23.8746, 19.5103) (-23.8829, 19.5152) (-23.8913, 19.5201) (-23.8997, 19.5251) (-23.9083, 19.5301) (-23.9169, 19.5352) (-23.9257, 19.5402) (-23.9345, 19.5453) (-23.9434, 19.5505) (-23.9525, 19.5556) (-23.9616, 19.5608) (-23.9708, 19.5661) (-23.9801, 19.5713) (-23.9895, 19.5766) (-23.999, 19.5819) (-24.0086, 19.5872) (-24.0182, 19.5926) (-24.028, 19.5979) (-24.0379, 19.6033) (-24.0478, 19.6088) (-24.0578, 19.6142) (-24.0679, 19.6197) (-24.0781, 19.6252) (-24.0884, 19.6307) (-24.0988, 19.6362) (-24.1092, 19.6417) (-24.1198, 19.6473) (-24.1304, 19.6529) (-24.1411, 19.6585) (-24.1519, 19.6641) (-24.1628, 19.6697) (-24.1737, 19.6754) (-24.1848, 19.6811) (-24.1959, 19.6867) (-24.2071, 19.6924) (-24.2184, 19.6981) (-24.2297, 19.7039) (-24.2412, 19.7096) (-24.2527, 19.7154) (-24.2643, 19.7211) (-24.276, 19.7269) (-24.2878, 19.7327) (-24.2996, 19.7385) (-24.3115, 19.7443) (-24.3235, 19.7501) (-24.3356, 19.7559) (-24.3478, 19.7618) (-24.36, 19.7676) (-24.3723, 19.7735) (-24.3847, 19.7793) (-24.3971, 19.7852) (-24.4097, 19.7911) (-24.4223, 19.797) (-24.435, 19.8029) (-24.4477, 19.8088) (-24.4606, 19.8147) (-24.4735, 19.8206) (-24.4865, 19.8265) (-24.4995, 19.8324) (-24.5126, 19.8383) (-24.5258, 19.8443) (-24.5391, 19.8502) (-24.5525, 19.8561) (-24.5659, 19.8621) (-24.5794, 19.868) (-24.5929, 19.874) (-24.6065, 19.8799) (-24.6202, 19.8859) (-24.634, 19.8918) (-24.6479, 19.8978) (-24.6618, 19.9037) (-24.6757, 19.9097) (-24.6898, 19.9156) (-24.7039, 19.9216) (-24.7181, 19.9275) (-24.7324, 19.9335) (-24.7467, 19.9395) (-24.7611, 19.9454) (-24.7755, 19.9514) (-24.7901, 19.9573) (-24.8046, 19.9633) (-24.8193, 19.9692) (-24.834, 19.9751) (-24.8488, 19.9811) (-24.8637, 19.987) (-24.8786, 19.993) (-24.8936, 19.9989) (-24.9087, 20.0048) (-24.9238, 20.0107) (-24.939, 20.0166) (-24.9542, 20.0226) (-24.9695, 20.0285) (-24.9849, 20.0344) (-25.0004, 20.0403) (-25.0159, 20.0462) (-25.0314, 20.052) (-25.0471, 20.0579) (-25.0628, 20.0638) (-25.0785, 20.0697) (-25.0943, 20.0755) (-25.1102, 20.0814) (-25.1262, 20.0872) (-25.1422, 20.0931) (-25.1583, 20.0989) (-25.1744, 20.1047) (-25.1906, 20.1105) (-25.2068, 20.1164) (-25.2232, 20.1222) (-25.2395, 20.1279) (-25.256, 20.1337) (-25.2725, 20.1395) (-25.289, 20.1453) (-25.3056, 20.151) (-25.3223, 20.1568) (-25.3391, 20.1625) (-25.3559, 20.1682) (-25.3727, 20.1739) (-25.3896, 20.1796) (-25.4066, 20.1853) (-25.4236, 20.191) (-25.4407, 20.1967) (-25.4579, 20.2023) (-25.4751, 20.208) (-25.4923, 20.2136) (-25.5097, 20.2192) (-25.527, 20.2248) (-25.5445, 20.2304) (-25.562, 20.236) (-25.5795, 20.2416) (-25.5971, 20.2471) (-25.6148, 20.2527) (-25.6325, 20.2582) (-25.6503, 20.2637) (-25.6681, 20.2693) (-25.686, 20.2747) (-25.7039, 20.2802) (-25.7219, 20.2857) (-25.74, 20.2911) (-25.7581, 20.2966) (-25.7763, 20.302) (-25.7945, 20.3074) (-25.8128, 20.3128) (-25.8311, 20.3182) (-25.8495, 20.3235) (-25.8679, 20.3289) (-25.8864, 20.3342) (-25.9049, 20.3395) (-25.9235, 20.3448) (-25.9422, 20.3501) (-25.9609, 20.3554) (-25.9796, 20.3606) (-25.9984, 20.3659) (-26.0173, 20.3711) (-26.0362, 20.3763) (-26.0552, 20.3815) (-26.0742, 20.3866) (-26.0933, 20.3918) (-26.1124, 20.3969) (-26.1316, 20.402) (-26.1508, 20.4071) (-26.1701, 20.4122) (-26.1894, 20.4173) (-26.2088, 20.4223) (-26.2282, 20.4273) (-26.2477, 20.4323) (-26.2672, 20.4373) (-26.2868, 20.4423) (-26.3064, 20.4472) (-26.3261, 20.4522) (-26.3459, 20.4571) (-26.3656, 20.462) (-26.3855, 20.4668) (-26.4054, 20.4717) (-26.4253, 20.4765) (-26.4453, 20.4813) (-26.4653, 20.4861) (-26.4854, 20.4909) (-26.5055, 20.4957) (-26.5257, 20.5004) (-26.5459, 20.5051) (-26.5662, 20.5098) (-26.5824, 20.5135) (-26.5946, 20.5163) (-26.6028, 20.5182) (-26.6069, 20.5191) knots 0 0 0 0 0 0 0.00416667 0.00833333 0.0125 0.01666667 0.02083333 0.025 0.02916667 0.03333333 0.0375 0.04166667 0.04583333 0.05 0.05416667 0.05833333 0.0625 0.06666667 0.07083333 0.075 0.07916667 0.08333333 0.0875 0.09166667 0.09583333 0.1 0.10416667 0.10833333 0.1125 0.11666667 0.12083333 0.125 0.12916667 0.13333333 0.1375 0.14166667 0.14583333 0.15 0.15416667 0.15833333 0.1625 0.16666667 0.17083333 0.175 0.17916667 0.18333333 0.1875 0.19166667 0.19583333 0.2 0.20416667 0.20833333 0.2125 0.21666667 0.22083333 0.225 0.22916667 0.23333333 0.2375 0.24166667 0.24583333 0.25 0.25416667 0.25833333 0.2625 0.26666667 0.27083333 0.275 0.27916667 0.28333333 0.2875 0.29166667 0.29583333 0.3 0.30416667 0.30833333 0.3125 0.31666667 0.32083333 0.325 0.32916667 0.33333333 0.3375 0.34166667 0.34583333 0.35 0.35416667 0.35833333 0.3625 0.36666667 0.37083333 0.375 0.37916667 0.38333333 0.3875 0.39166667 0.39583333 0.4 0.40416667 0.40833333 0.4125 0.41666667 0.42083333 0.425 0.42916667 0.43333333 0.4375 0.44166667 0.44583333 0.45 0.45416667 0.45833333 0.4625 0.46666667 0.47083333 0.475 0.47916667 0.48333333 0.4875 0.49166667 0.49583333 0.5 0.50416667 0.50833333 0.5125 0.51666667 0.52083333 0.525 0.52916667 0.53333333 0.5375 0.54166667 0.54583333 0.55 0.55416667 0.55833333 0.5625 0.56666667 0.57083333 0.575 0.57916667 0.58333333 0.5875 0.59166667 0.59583333 0.6 0.60416667 0.60833333 0.6125 0.61666667 0.62083333 0.625 0.62916667 0.63333333 0.6375 0.64166667 0.64583333 0.65 0.65416667 0.65833333 0.6625 0.66666667 0.67083333 0.675 0.67916667 0.68333333 0.6875 0.69166667 0.69583333 0.7 0.70416667 0.70833333 0.7125 0.71666667 0.72083333 0.725 0.72916667 0.73333333 0.7375 0.74166667 0.74583333 0.75 0.75416667 0.75833333 0.7625 0.76666667 0.77083333 0.775 0.77916667 0.78333333 0.7875 0.79166667 0.79583333 0.8 0.80416667 0.80833333 0.8125 0.81666667 0.82083333 0.825 0.82916667 0.83333333 0.8375 0.84166667 0.84583333 0.85 0.85416667 0.85833333 0.8625 0.86666667 0.87083333 0.875 0.87916667 0.88333333 0.8875 0.89166667 0.89583333 0.9 0.90416667 0.90833333 0.9125 0.91666667 0.92083333 0.925 0.92916667 0.93333333 0.9375 0.94166667 0.94583333 0.95 0.95416667 0.95833333 0.9625 0.96666667 0.97083333 0.975 0.97916667 0.98333333 0.9875 0.99166667 0.99583333 1 1 1 1 1 1
  arc A55 (-26.6069, 20.5191) -> (-27.7368, 18.9639) centre (0, 0) ccw